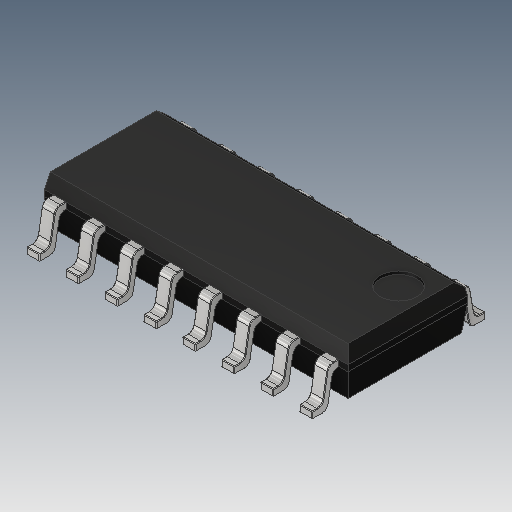
# Autodesk Inventor part: SOP-16
Saved by Autodesk Inventor 2017 (Build 210142000, 142)
## iProperties
Created: 2016-06-28
Part Number: SOP-16
Material: Generic
Document SubType Name: Modeling
Designer: Jonathan
Density: 1 g/cm^3
Appearance: Default
Author: Jonathan
Autodesk Inventor part; units mm, degrees
ref_plane "YZ Plane" through (0, 0, 0) normal (1, 0, 0) x (0, 1, 0)
sketch "Sketch1" plane through (0, 0, 0) normal (0, 1, 0) x (-1, 0, 0)
  line L0 (4.95, -1.95) -> (-4.95, -1.95)
  line L1 (-4.95, -1.95) -> (-4.95, 1.95)
  line L2 (-4.95, 1.95) -> (4.95, 1.95)
  line L3 (4.95, 1.95) -> (4.95, -1.95)
  point P0 (0, 0)
  point P1 (0, -1.95)
  point P2 (-4.95, 0)
  dimension "d0" = 9.9
  dimension "d1" = 3.9
  constraints: 8 end point, 2 midpoint, 2 parallel, 1 horizontal, 1 horizontal alignment, 1 perpendicular, 1 vertical alignment
  measures "d0" distance of L0.start L0.end
  measures "d1" distance of L0.end L1.end
extrude "Extrusion1" add sketch "Sketch1" along normal blind 1.55
sketch "Sketch4" plane through (-4.95, 0, 1.95) normal (0, 0, 1) x (1, 0, 0)
  line L0 (9.185, 1.06) -> (9.605, 1.06)
  line L1 (9.605, 1.06) -> (9.605, 0.84)
  line L2 (9.605, 0.84) -> (9.185, 0.84)
  line L3 (9.185, 0.84) -> (9.185, 1.06)
  line L4 (9.9, 1.55) -> (0, 1.55) projected
  line L5 (9.185, 1.06) -> (9.605, 0.84) construction
  line L6 (9.605, 1.06) -> (9.185, 0.84) construction
  line L7 (9.9, 0) -> (9.9, 1.55) projected
  point P0 (4.95, 0)
  point P1 (9.395, 0.95)
  dimension "d25" = 0.42
  dimension "d26" = 0.22
  dimension "d28" = 0.6
  dimension "d29" = 0.505
  constraints: 12 end point, 2 parallel, 1 horizontal, 1 midpoint, 1 perpendicular
  measures "d25" distance of L0.start L0.end
  measures "d26" distance of L0.end L1.end
  measures "d28" distance from line of L4 point (9.395, 0.95)
  measures "d29" distance from line of L7 point (9.395, 0.95)
extrude "Extrusion2" add sketch "Sketch4" along normal blind 0.35 separate body
ref_plane "Work Plane2" through (4.235, 1.06, 2.3) normal (0, 0.9848078, -0.1736482) x (-1, 0, 0)
sketch "Sketch6" plane through (4.235, 1.06, 2.3) normal (0, 0.9848078, -0.1736482) x (-1, 0, 0)
  line L0 (-0.42, -0.3829) -> (-0.42, -0.0382) projected
  line L1 (0, 0) -> (-0.42, 0)
  line L2 (-0.42, 0) -> (-0.42, -0.2)
  line L3 (-0.42, -0.2) -> (0, -0.2)
  line L4 (0, -0.2) -> (0, 0)
  line L5 (-0.42, 0) -> (0, 0) projected
  line L6 (0, 0) -> (0, -0.0382) projected
  point P0 (4.235, -2.4491)
  dimension "d33" = 0.2
  constraints: 8 end point, 2 parallel, 2 point on line, 1 collinear, 1 horizontal, 1 perpendicular
  measures "d33" distance of L1.end L2.end
extrude "Extrusion3" add sketch "Sketch6" against normal blind 1.25 bodies 2
ref_plane "Work Plane3" through (4.655, -0.2057, 2.3201) normal (0, 0, 1) x (1, 0, 0)
sketch "Sketch7" plane through (4.655, -0.2057, 2.3201) normal (0, 0, 1) x (1, 0, 0)
  line L0 (-0.42, 0) -> (0, 0) projected
  line L1 (-0.42, 1.0457) -> (-0.42, 0) projected
  line L2 (0, 0) -> (-0.42, 0)
  line L3 (-0.42, 0) -> (-0.42, 0.22)
  line L4 (-0.42, 0.22) -> (0, 0.22)
  line L5 (0, 0.22) -> (0, 0)
  point P0 (-4.655, 0.2057)
  point P1 (-0.42, 1.231)
  dimension "d36" = 0.22
  constraints: 8 end point, 2 parallel, 1 horizontal, 1 perpendicular, 1 point on line
  measures "d36" distance of L4.end L0.end
extrude "Extrusion4" add sketch "Sketch7" along normal blind 0.5 bodies 2
fillet "Fillet3" radius 0.2 4 edges at (4.445, 1.06, 2.3) (4.445, 0.0143, 2.4844) (4.445, -0.2057, 2.3201) (4.445, 0.84, 2.1357)
fillet "Fillet4" radius 0.02 24 edges at (4.655, 0.0611, 2.5237) (4.655, 0.0143, 2.7362) (4.655, 1.0132, 2.2607) (4.655, 1.06, 2.0411) (4.655, 0.5371, 2.3922) (4.235, 0.0611, 2.5237) (4.235, 0.0143, 2.7362) (4.235, 1.0132, 2.2607) (4.235, 1.06, 2.0411) (4.235, 0.5371, 2.3922) (4.655, -0.1589, 2.3594) (4.655, -0.2057, 2.654) (4.655, 0.7932, 2.0964) (4.655, 0.84, 1.9589) (4.655, 0.3171, 2.2279) (4.235, -0.1589, 2.3594) (4.235, 0.3171, 2.2279) (4.235, 0.7932, 2.0964) (4.235, 0.84, 1.9589) (4.235, -0.2057, 2.654) (4.445, 0.0143, 2.8201) (4.235, -0.0957, 2.8201) (4.445, -0.2057, 2.8201) (4.655, -0.0957, 2.8201)
pattern_linear "Rectangular Pattern2" count 8 spacing 1.27 along (-1, 0, 0) of "Extrusion2", "Extrusion3", "Extrusion4", "Fillet3", "Fillet4" bodies 2
mirror "Mirror1" about plane through (0, 0, 0) normal (0, 0, 1) of "Extrusion2", "Extrusion3", "Extrusion4", "Fillet3", "Fillet4", "Rectangular Pattern2" bodies 2
chamfer "Chamfer1" distance 0.1 distance2 0.5 1 edges at (4.95, 1.55, 0) measured on face at (4.45, 1.55, 0)
chamfer "Chamfer2" distance 0.1 distance2 0.5 1 edges at (-4.95, 1.55, 0) measured on face at (-4.45, 1.55, 0)
chamfer "Chamfer3" distance 0.1 distance2 0.85 1 edges at (4.95, 0, 0) measured on face at (4.45, 0, 0)
chamfer "Chamfer4" distance 0.1 distance2 0.85 1 edges at (-4.95, 0, 0) measured on face at (-4.45, 0, 0)
chamfer "Chamfer5" distance 0.1 distance2 0.85 1 edges at (0, 0, -1.95) measured on face at (0, 0, -1.45)
chamfer "Chamfer6" distance 0.1 distance2 0.85 1 edges at (0, 0, 1.95) measured on face at (0, 0, 1.45)
chamfer "Chamfer7" distance 0.1 distance2 0.5 1 edges at (0, 1.55, 1.95) measured on face at (0, 1.55, 1.45)
chamfer "Chamfer8" distance 0.1 distance2 0.5 1 edges at (0, 1.55, -1.95) measured on face at (0, 1.55, -1.45)
chamfer "Chamfer9" distance 0.25 distance2 0.25 1 edges at (0, 1.55, -1.85) measured on face at (0, 1.4519, -1.8696)
sketch "Sketch8" plane through (0, 1.55, 0) normal (0, 1, 0) x (1, 0, 0)
  circle A0 centre (4.05, 0.6) radius 0.6
  line L0 (-4.85, 1.6) -> (4.85, 1.6) projected
  line L1 (4.85, 1.6) -> (4.85, -1.85) projected
  point P0 (0, 0)
  dimension "d76" = 1
  dimension "d77" = 0.8
  dimension "d78" = 1.2
  constraints: 1 centre point
  measures "d76" distance from line of L0 A0.centre
  measures "d77" distance from line of L1 A0.centre
  measures "d78" diameter of A0
extrude "Extrusion5" cut sketch "Sketch8" against normal blind 0.1 bodies 1
body "Solid1"
body "Solid2"
